simple_wafer_v1 (Autodesk Fusion 360 design; units mm, degrees)
Autodesk Fusion 360 part; units mm, degrees
cylinder "CylinderPrimitive1" add diameter 101.6 height 0.2 placed x (1, 0, 0) y (0, 0, -1) z (0, 1, 0) at (0, 0, 0)
